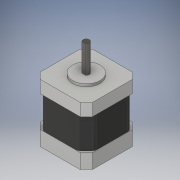
# Autodesk Inventor part: 42BYGH47
Saved by Autodesk Inventor 2019 (Build 230136000, 136)
## iProperties
Created: 2020-12-05
Part Number: 42BYGH47
Material: Сталь, мягкая
Document SubType Name: Modeling
Designer: Professional
Density: 7.85 g/cm^3
Appearance: С умеренной полировкой
Author: Professional
Autodesk Inventor part; units mm, degrees
ref_plane "YZ Plane" through (0, 0, 0) normal (1, 0, 0) x (0, 1, 0)
ref_plane "XZ Plane" through (0, 0, 0) normal (0, 1, 0) x (-1, 0, 0)
ref_plane "XY Plane" through (0, 0, 0) normal (0, 0, 1) x (1, 0, 0)
sketch "Эскиз1" plane through (0, 0, 0) normal (0, 1, 0) x (-1, 0, 0)
  line L0 (16.15, 21.15) -> (-16.15, 21.15)
  line L1 (-21.15, 16.15) -> (-21.15, -16.15)
  line L2 (-16.15, -21.15) -> (16.15, -21.15)
  line L3 (21.15, -16.15) -> (21.15, 16.15)
  line L4 (21.15, 21.15) -> (-21.15, -21.15) construction
  line L5 (-21.15, 21.15) -> (21.15, -21.15) construction
  line L6 (16.15, -21.15) -> (21.15, -16.15)
  line L7 (21.15, 16.15) -> (16.15, 21.15)
  line L8 (-16.15, 21.15) -> (-21.15, 16.15)
  line L9 (-21.15, -16.15) -> (-16.15, -21.15)
  point P0 (0, 0)
  dimension "d0" = 42.3
  dimension "d1" = 5
  dimension "d2" = 5
  dimension "d3" = 5
  dimension "d4" = 5
  dimension "d5" = 5
  dimension "d6" = 5
  dimension "d7" = 5
  dimension "d8" = 5
  constraints: 20 end point, 8 point on line, 2 midpoint, 2 parallel, 2 perpendicular, 1 horizontal
  measures "d0" distance between parallel lines of L0 L2
  measures "d1" distance of L2.end L5.end
  measures "d2" distance of L3.start L5.end
  measures "d3" distance of L3.end L4.start
  measures "d4" distance of L0.start L4.start
  measures "d5" distance of L0.end L5.start
  measures "d6" distance of L1.start L5.start
  measures "d7" distance of L1.end L4.end
  measures "d8" distance of L2.start L4.end
extrude "Выдавливание1" add sketch "Эскиз1" along normal blind 12
sketch "Эскиз2" plane through (0, 12, 0) normal (0, 1, 0) x (1, 0, 0)
  line L0 (13.95, -20.95) -> (-13.95, -20.95)
  line L1 (-20.95, -13.95) -> (-20.95, 13.95)
  line L2 (-13.95, 20.95) -> (13.95, 20.95)
  line L3 (20.95, 13.95) -> (20.95, -13.95)
  line L4 (20.95, -20.95) -> (-20.95, 20.95) construction
  line L5 (-20.95, -20.95) -> (20.95, 20.95) construction
  line L6 (-16.15, -21.15) -> (16.15, -21.15) projected
  line L7 (-13.95, -20.95) -> (-20.95, -13.95)
  line L8 (-20.95, 13.95) -> (-13.95, 20.95)
  line L9 (13.95, 20.95) -> (20.95, 13.95)
  line L10 (20.95, -13.95) -> (13.95, -20.95)
  point P0 (0, 0)
  dimension "d23" = 0.2
  dimension "d24" = 7
  dimension "d25" = 7
  dimension "d26" = 7
  dimension "d27" = 7
  dimension "d28" = 7
  dimension "d29" = 7
  dimension "d30" = 7
  dimension "d31" = 7
  constraints: 20 end point, 8 point on line, 2 midpoint, 2 parallel, 2 perpendicular, 1 horizontal
  measures "d23" distance between parallel lines of L6 L0
  measures "d24" distance of L0.end L5.start
  measures "d25" distance of L1.start L5.start
  measures "d26" distance of L1.end L4.end
  measures "d27" distance of L2.start L4.end
  measures "d28" distance of L2.end L5.end
  measures "d29" distance of L3.start L5.end
  measures "d30" distance of L3.end L4.start
  measures "d31" distance of L0.start L4.start
extrude "Выдавливание2" add sketch "Эскиз2" along normal blind 25
sketch "Эскиз3" plane through (0, 37, 0) normal (0, 1, 0) x (1, 0, 0)
  line L0 (-16.15, 21.15) -> (-21.15, 16.15) projected
  line L1 (16.15, 21.15) -> (-16.15, 21.15) projected
  line L2 (21.15, 16.15) -> (16.15, 21.15) projected
  line L3 (21.15, -16.15) -> (21.15, 16.15) projected
  line L4 (16.15, -21.15) -> (21.15, -16.15) projected
  line L5 (-16.15, -21.15) -> (16.15, -21.15) projected
  line L6 (-21.15, -16.15) -> (-16.15, -21.15) projected
  line L7 (-21.15, 16.15) -> (-21.15, -16.15) projected
  point P0 (0, 0)
extrude "Выдавливание3" add sketch "Эскиз3" along normal blind 10
fillet "Сопряжение1" radius 3 8 edges at (13.95, 24.5, 20.95) (20.95, 24.5, 13.95) (20.95, 24.5, -13.95) (13.95, 24.5, -20.95) (-13.95, 24.5, -20.95) (-20.95, 24.5, -13.95) (-20.95, 24.5, 13.95) (-13.95, 24.5, 20.95)
sketch "Эскиз4" plane through (0, 47, 0) normal (0, 1, 0) x (1, 0, 0)
  circle A0 centre (0, 0) radius 11
  dimension "d33" = 22
  constraints: 1 centre point, 1 coincident
  measures "d33" diameter of A0
extrude "Выдавливание4" add sketch "Эскиз4" along normal blind 2
sketch "Эскиз5" plane through (0, 49, 0) normal (0, 1, 0) x (1, 0, 0)
  arc A0 (1.5, -2) -> (-1.5, -2) centre (0, 0) ccw
  line L0 (1.5, -2) -> (-1.5, -2)
  dimension "d36" = 2.5
  dimension "d37" = 2
  constraints: 2 end point, 2 point on circle, 1 centre point, 1 coincident, 1 horizontal
  measures "d36" radius of A0
  measures "d37" distance from line of point (0, 0) L0
extrude "Выдавливание5" add sketch "Эскиз5" along normal blind 22
sketch "Эскиз6" plane through (16.15, 0, -21.15) normal (0, 0, -1) x (-1, 0, 0)
  line L0 (0, 0) -> (32.3, 0) projected
  line L1 (8.65, 11) -> (23.65, 11)
  line L2 (23.65, 11) -> (23.65, 5)
  line L3 (23.65, 5) -> (8.65, 5)
  line L4 (8.65, 5) -> (8.65, 11)
  point P0 (16.15, 0)
  point P1 (16.15, 0)
  point P2 (16.15, 5)
  point P3 (16.15, 0)
  dimension "d67" = 15
  dimension "d68" = 6
  dimension "d69" = 5
  constraints: 8 end point, 3 midpoint, 2 parallel, 1 horizontal, 1 perpendicular, 1 vertical alignment
  measures "d67" distance of L2.end L3.end
  measures "d68" distance of L1.end L2.end
  measures "d69" distance between parallel lines of L0 L3
extrude "Выдавливание6" add sketch "Эскиз6" along normal blind 6
sketch "Эскиз9" plane through (16.15, 0, -27.15) normal (0, 0, -1) x (-1, 0, 0)
  line L0 (9.15, 10.5) -> (23.15, 10.5)
  line L1 (23.15, 10.5) -> (23.15, 6.5)
  line L2 (23.15, 6.5) -> (9.15, 6.5)
  line L3 (9.15, 6.5) -> (9.15, 10.5)
  line L4 (23.65, 5) -> (23.65, 11) projected
  line L5 (23.65, 11) -> (8.65, 11) projected
  point P0 (16.15, 0)
  point P1 (16.15, 6.5)
  dimension "d70" = 0.5
  dimension "d71" = 0.5
  dimension "d72" = 4
  constraints: 8 end point, 2 parallel, 1 horizontal, 1 midpoint, 1 perpendicular, 1 vertical alignment
  measures "d70" distance between parallel lines of L4 L1
  measures "d71" distance between parallel lines of L5 L0
  measures "d72" distance between parallel lines of L2 L0
extrude "Выдавливание8" cut sketch "Эскиз9" against normal blind 4
chamfer "Фаска1" distance 0.5 angle 45 4 edges at (7.5, 11, -24.15) (7.5, 5, -24.15) (-7.5, 11, -24.15) (-7.5, 5, -24.15)
equation "\"d2\" = d1"
equation "\"d3\" = d1"
equation "\"d4\" = d3"
equation "\"d5\" = d1"
equation "\"d6\" = d5"
equation "\"d7\" = d1"
equation "\"d8\" = d7"
equation "\"d25\" = d24"
equation "\"d26\" = d24"
equation "\"d27\" = d26"
equation "\"d28\" = d24"
equation "\"d29\" = d28"
equation "\"d30\" = d24"
equation "\"d31\" = d30"
